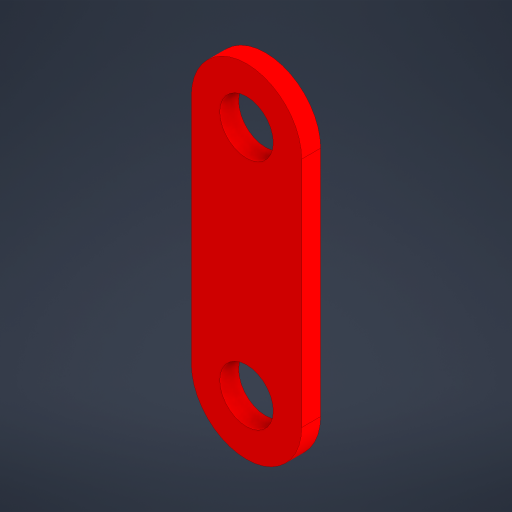
# Autodesk Inventor part: not flex back qre flex holder
Saved by Autodesk Inventor 2024 (Build 280153000, 153)
## iProperties
Created: 2024-03-06
Part Number: not flex back qre flex holder
Material: Všeobecné
Document SubType Name: Modeling
Designer: Simak
Density: 1 g/cm^3
Appearance: Výchozí
Author: Simak
Autodesk Inventor part; units mm, degrees
ref_plane "YZ Plane" through (0, 0, 0) normal (1, 0, 0) x (0, 1, 0)
ref_plane "XZ Plane" through (0, 0, 0) normal (0, 1, 0) x (-1, 0, 0)
ref_plane "XY Plane" through (0, 0, 0) normal (0, 0, 1) x (1, 0, 0)
sketch "Náčrt1" plane through (0, 0, 0) normal (0, 0, 1) x (1, 0, 0)
  line L0 (0, 7.375) -> (0, -7.375) construction
  line L1 (-3.5, 7.375) -> (-3.5, -7.375)
  line L2 (3.5, -7.375) -> (3.5, 7.375)
  arc A0 (3.5, 7.375) -> (-3.5, 7.375) centre (0, 7.375) ccw
  arc A1 (-3.5, -7.375) -> (3.5, -7.375) centre (0, -7.375) ccw
  circle A2 centre (0, 7.375) radius 1.7
  circle A3 centre (0, -7.375) radius 1.7
  circle A4 centre (0, 7.375) radius 3.5
  point P0 (0, 0)
  point P1 (0, 0)
  point P2 (-3.5, 7.375)
  point P3 (3.5, 7.375)
  dimension "d0" = 14.75
  dimension "d1" = 3.5
  dimension "d2" = 3.4
  constraints: 8 end point, 5 centre point, 4 coincident, 4 point on circle, 4 tangent, 2 equal radius, 1 midpoint, 1 parallel, 1 vertical
  measures "d0" distance of L0.end L0.start
  measures "d1" radius of A0
  measures "d2" diameter of A2
extrude "Vysunutí1" add sketch "Náčrt1" along normal blind 1.2
